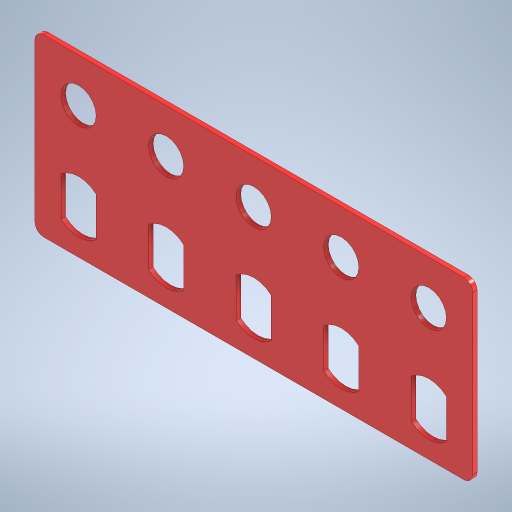
# Autodesk Inventor part: 1020
Saved by Autodesk Inventor 2024 (Build 280153000, 153)
## iProperties
Created: 2024-09-20
Part Number: 1020
Material: Všeobecné
Document SubType Name: Modeling
Designer: Student
Density: 1 g/cm^3
Appearance: Světle červená
Author: Student
Autodesk Inventor part; units mm, degrees
ref_plane "YZ Plane" through (0, 0, 0) normal (1, 0, 0) x (0, 1, 0)
ref_plane "XZ Plane" through (0, 0, 0) normal (0, 1, 0) x (-1, 0, 0)
ref_plane "XY Plane" through (0, 0, 0) normal (0, 0, 1) x (1, 0, 0)
sketch "Náčrt1" plane through (0, 0, 0) normal (0, 0, 1) x (1, 0, 0)
  line L0 (-40, 10) -> (10, 10)
  line L1 (10, 10) -> (10, -10)
  line L2 (10, -10) -> (-40, -10)
  line L3 (-40, -10) -> (-40, 10)
  point P0 (0, 0)
  dimension "d0" = 20
  dimension "d1" = 50
  dimension "d2" = 10
  dimension "d3" = 10
  constraints: 8 end point, 2 parallel, 1 horizontal, 1 perpendicular
  measures "d0" distance between parallel lines of L2 L0
  measures "d1" distance between parallel lines of L3 L1
  measures "d2" distance from line of L1 point (0, 0)
  measures "d3" distance from line of L0 point (0, 0)
extrude "Vysunutí1" add sketch "Náčrt1" along normal blind 0.5
sketch "Náčrt2" plane through (0, 0, 0.5) normal (0, 0, 1) x (1, 0, 0)
  circle A0 centre (-35, 5) radius 2
  line L0 (10, 10) -> (-40, 10) projected
  line L1 (-40, 10) -> (-40, -10) projected
  point P0 (0, 0)
  dimension "d6" = 4
  dimension "d7" = 5
  dimension "d8" = 5
  constraints: 1 centre point
  measures "d6" diameter of A0
  measures "d7" distance from line of L0 A0.centre
  measures "d8" distance from line of L1 A0.centre
extrude "Vysunutí2" cut sketch "Náčrt2" against normal blind 0.5
pattern_linear "Obdélníkové pole1" count 7 spacing 10 along (1, 0, 0) of "Vysunutí2"
fillet "Zaoblení1" radius 1 1 edges at (10, 10, 0.25)
fillet "Zaoblení2" radius 1 2 edges at (-40, 10, 0.25) (-40, -10, 0.25)
fillet "Zaoblení3" radius 1 1 edges at (10, -10, 0.25)
sketch "Náčrt3" plane through (0, 0, 0.5) normal (0, 0, 1) x (1, 0, 0)
  line L0 (7, -2.7639) -> (7, -7.2361)
  line L1 (3, -2.7639) -> (3, -7.2361)
  arc A0 (7, -2.7639) -> (3, -2.7639) centre (5, -5) ccw
  arc A1 (3, -7.2361) -> (7, -7.2361) centre (5, -5) ccw
  line L2 (10, -9) -> (10, 9) projected
  line L3 (-39, -10) -> (9, -10) projected
  point P0 (0, 0)
  point P1 (3, -7.229)
  point P2 (5, -8)
  point P3 (5, -2)
  dimension "d24" = 2
  dimension "d25" = 4
  dimension "d26" = 5
  dimension "d27" = 5
  dimension "d28" = 3
  dimension "d29" = 3
  constraints: 6 point on circle, 4 end point, 2 centre point, 1 point on line
  measures "d24" distance from line of A0.centre L0
  measures "d25" distance from line of point (3, -7.229) L0
  measures "d26" distance from line of L2 A0.centre
  measures "d27" distance from line of L3 A0.centre
  measures "d28" distance of A0.centre point (5, -8)
  measures "d29" distance of A0.centre point (5, -2)
extrude "Vysunutí3" cut sketch "Náčrt3" against normal blind 10
pattern_linear "Obdélníkové pole2" count 7 spacing 10 along (-1, 0, 0) of "Vysunutí3"
